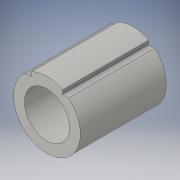
# Autodesk Inventor part: Nathan_RobotArm_TwistPart
Saved by Autodesk Inventor 2016 (Build 200138000, 138)
## iProperties
Created: 2017-03-30
Part Number: Nathan_RobotArm_TwistPart
Material: Generic
Document SubType Name: Modeling
Designer: brandn
Density: 1 g/cm^3
Appearance: Default
Author: brandn
Autodesk Inventor part; units mm, degrees
ref_plane "YZ Plane" through (0, 0, 0) normal (1, 0, 0) x (0, 1, 0)
ref_plane "XZ Plane" through (0, 0, 0) normal (0, 1, 0) x (-1, 0, 0)
ref_plane "XY Plane" through (0, 0, 0) normal (0, 0, 1) x (1, 0, 0)
sketch "Sketch1" plane through (0, 0, 0) normal (0, 0, 1) x (1, 0, 0)
  circle A0 centre (0, 0) radius 13.335
  circle A1 centre (0, 0) radius 19.685
  dimension "d0" = 26.67
  dimension "d1" = 39.37
  constraints: 2 centre point, 2 coincident
  measures "d0" diameter of A0
  measures "d1" diameter of A1
extrude "Extrusion1" add sketch "Sketch1" along normal blind 50.8
sketch "Sketch2" plane through (0, 0, 50.8) normal (0, 0, 1) x (1, 0, 0)
  line L0 (-12.9952, 15.0174) -> (-9.1852, 15.0174)
  line L1 (-9.1852, 15.0174) -> (-9.1852, 19.9304)
  line L2 (-9.1852, 19.9304) -> (-12.9952, 19.9304)
  line L3 (-12.9952, 19.9304) -> (-12.9952, 15.0174)
  circle A0 centre (0, 0) radius 19.685 projected
  line L4 (9.2044, 15.0174) -> (13.0144, 15.0174)
  line L5 (13.0144, 15.0174) -> (13.0144, 20.792)
  line L6 (13.0144, 20.792) -> (9.2044, 20.792)
  line L7 (9.2044, 20.792) -> (9.2044, 15.0174)
  point P0 (0.0096, 19.685)
  dimension "d4" = 3.81
  dimension "d5" = 9.1948
  dimension "d6" = 3.81
  dimension "d7" = 9.1948
  constraints: 16 end point, 4 parallel, 2 horizontal, 2 perpendicular, 2 other
  measures "d4" distance of L2.end L1.end
  measures "d5" distance from line of L1 point (0.01, 19.685)
  measures "d6" distance of L6.end L5.end
  measures "d7" distance from line of point (0.01, 19.685) L7
extrude "Extrusion2" cut sketch "Sketch2" against normal blind 50.8 contours L3 L2 L1 A0 L0 | A0 L1 L0 | L7 L6 L5 L4 A0 | A0 L4 L7
body "Solid1"
